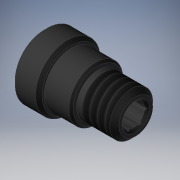
# Autodesk Inventor part: VPM46-6
Saved by Autodesk Inventor 2019 (Build 230136000, 136)
## iProperties
Created: 2023-10-05
Part Number: VPM46-6
Material: Generic
Catalog Web Link: www.cadenas.de
Description: VPM-Pad screw
Vendor: PISCO_JP
Document SubType Name: Modeling
Designer: psAdmin
Manufacturer: PISCO_JP
Mass: 0.10567 g
Surface Area: 2.4069 cm^2
Volume: 0.10567 cm^3
Density: 1 g/cm^3
Appearance: PSOLRGB-175-175-175
Category: PARTsolutions
Company: PISCO_JP
Title: VPM46-6
Author: Cadenas PARTsolutions
Comments: Pad screw
PSOL_IDENT_0: {$CADENAS_DATA/23d-libs/pisco_jp/vacuum_pad_series_r2/vacuum_pad_pad_and_holder_joint_assy/commonpoo
PSOL_IDENT_1: l/pad_screw.prj},151 {VTYP=3D},{NB=VPM46-6},{LINA=VPM46-6},{NN=VPM},{DATE=05.10.2020 07:46:03},{GEOM
PSOL_IDENT_2: DATE=08.01.2020 12:32:14},{VERSION=},{LINEID=10},{WBVAR=},{WBNUMERIC=}  {NB=VPM46-6},{LINA=VPM46-6},
PSOL_IDENT_3: {KT=DUMMY},{CNSORDERNO=VPM46-6},{M=-},{NDM=0.000},{PITCH=0.000},{D=0.000},{SD=0.000},{P=0.000},{E=0.
PSOL_IDENT_4: 000},{A=0.000},{C=0.000},{B=0.000},{L1=0.000},{L2=0.000},{HEX=0.000},{VER=1}
NB: VPM46-6
NN: VPM
NT: Pad screw
NBSYN: $CNSORDERNO.
LINA: VPM46-6
CATALOG: NIHON PISCO CO., LTD
CNSORDERNO: VPM46-6
M: -
NDM: 0
PITCH: 0
D: 0
SD: 0
P: 0
E: 0
A: 0
C: 0
B: 0
L1: 0
L2: 0
HEX: 0
VER: 1
SUPPLIER: PISCO_JP
ARTICLENO: VPM46-6
BOMINFO: VPM46-6
CREATOR: CADENAS GmbH
Autodesk Inventor part; units mm, degrees
sketch "Sketch_1" plane through (0, 0, 0) normal (0, 0, 1) x (1, 0, 0)
  line L0 (8.5, 0) -> (0, 0)
  line L1 (0, 0) -> (0, 2.7)
  line L2 (0, 2.7) -> (0.3, 3)
  line L3 (0.3, 3) -> (2.2, 3)
  line L4 (2.2, 3) -> (2.5, 2.7)
  line L5 (2.5, 2.7) -> (2.5, 2.5)
  line L6 (2.5, 2.5) -> (4.8, 2.5)
  line L7 (4.8, 2.5) -> (5, 2.3)
  line L8 (5, 2.3) -> (5, 2)
  line L9 (5, 2) -> (8.0705, 2)
  line L10 (8.0705, 2) -> (8.5, 1.5705)
  line L11 (8.5, 1.5705) -> (8.5, 0)
  line L12 (8.5, 0) -> (0, 0)
  constraints: 26 end point
revolve "Revolution1" add sketch "Sketch_1" angle 360 about axis through (8.5, 0, 0) along (1, 0, 0)
thread "Thread1" size "M4x0.7" class "6g" standard "ISO Metric profile" length 2.5705
sketch "Sketch_2" plane through (0, 0, 0) normal (0, 0, 1) x (1, 0, 0)
  line L0 (8.5, 0) -> (0, 0)
  line L1 (0, 0) -> (0, 1.85)
  line L2 (0, 1.85) -> (0.1, 1.75)
  line L3 (0.1, 1.75) -> (4, 1.75)
  line L4 (4, 1.75) -> (4, 1.29)
  line L5 (4, 1.29) -> (4.24, 1.05)
  line L6 (4.24, 1.05) -> (8.26, 1.05)
  line L7 (8.26, 1.05) -> (8.5, 1.29)
  line L8 (8.5, 1.29) -> (8.5, 0)
  line L9 (8.5, 0) -> (0, 0)
  constraints: 20 end point
revolve "Revolution2" cut sketch "Sketch_2" angle 360 about axis through (8.5, 0, 0) along (1, 0, 0)
sketch "Sketch_3" plane through (8.5, 0, 0) normal (1, 0, 0) x (0, 1, 0)
  line L0 (-1, -0.5774) -> (0, -1.1547)
  line L1 (0, -1.1547) -> (1, -0.5774)
  line L2 (1, -0.5774) -> (1, 0.5774)
  line L3 (1, 0.5774) -> (0, 1.1547)
  line L4 (0, 1.1547) -> (-1, 0.5774)
  line L5 (-1, 0.5774) -> (-1, -0.5774)
  constraints: 12 end point
extrude "Extrusion1" cut sketch "Sketch_3" against normal blind 4.5
ref_plane "IP_screw_XY" through (2.5, 0, 0) normal (1, 0, 0) x (0, 0, -1)
ref_plane "IP_screw_YZ" through (2.5, 0, 0) normal (0, 0, -1) x (0, 1, 0)
ref_plane "IP_screw_ZX" through (2.5, 0, 0) normal (0, 1, 0) x (1, 0, 0)
body "Solid1"
